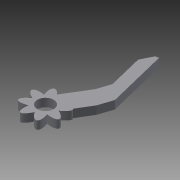
# Autodesk Inventor part: BrazoPinza
Saved by Autodesk Inventor 2015 (Build 190159000, 159)
## iProperties
Created: 2013-11-10
Part Number: BrazoPinza
Material: Genérico
Document SubType Name: Modeling
Designer: Gregorio
Density: 1 g/cm^3
Appearance: Valor por defecto
Author: Gregorio
Autodesk Inventor part; units mm, degrees
ref_plane "YZ Plane" through (0, 0, 0) normal (1, 0, 0) x (0, 1, 0)
ref_plane "XZ Plane" through (0, 0, 0) normal (0, 1, 0) x (-1, 0, 0)
ref_plane "XY Plane" through (0, 0, 0) normal (0, 0, 1) x (1, 0, 0)
sketch "Boceto1" plane through (0, 0, 0) normal (0, 0, 1) x (1, 0, 0)
  circle A0 centre (0, 0) radius 12.5
  circle A1 centre (0, 0) radius 4
  ellipse E0 centre (0, 4) end of major axis (0, 12.5) minor radius 3
  ellipse E1 centre (2.85, 2.8067) end of major axis (8.9175, 8.7595) minor radius 3
  ellipse E2 centre (4, 0) end of major axis (12.5, 0) minor radius 3
  ellipse E3 centre (2.85, -2.8067) end of major axis (8.8031, -8.8744) minor radius 3
  ellipse E4 centre (0, -4) end of major axis (0, -12.5) minor radius 3
  ellipse E5 centre (-2.85, -2.8067) end of major axis (-8.9175, -8.7595) minor radius 3
  ellipse E6 centre (-4, 0) end of major axis (-12.5, 0) minor radius 3
  ellipse E7 centre (-2.85, 2.8067) end of major axis (-8.8031, 8.8744) minor radius 3
  dimension "d1" = 8
  dimension "d4" = 3
  dimension "d5" = 3
  dimension "d6" = 3
  dimension "d7" = 3
  dimension "d8" = 3
  dimension "d9" = 3
  dimension "d10" = 3
  dimension "d11" = 3
  dimension "d0" = 25
  dimension "d12" = 2.85
  dimension "d14" = 2.85
  dimension "d15" = 2.85
  dimension "d16" = 2.85
  constraints: 2 coincident, 2 horizontal alignment, 2 vertical alignment, 1 centre point, 34 other
  measures "d0" diameter of A0
  measures "d12" horizontal distance of point (2.85, 2.807) point (0, 4)
  measures "d14" horizontal distance of point (-2.85, 2.807) point (0, 4)
  measures "d15" horizontal distance of point (0, -4) point (-2.85, -2.807)
  measures "d16" horizontal distance of point (2.85, -2.807) point (0, -4)
extrude "Extrusión1" add sketch "Boceto1" along normal blind 2 contours E2 E3 E6 E1 | E1 E2 E5 E0 | E3 E4 E7 E2 | E1 E6 A1 E5 E2 | E2 E7 A1 E6 E3 | E0 E1 E4 E7 | E0 E5 A1 E4 E1 | E4 E5 E0 E3 | E3 E0 A1 E7 E4 | E6 E3 E1 | E1 E3 A1 E6 | E5 A1 E0 E2 | E2 E0 E5 | E7 E4 E2 | E2 E4 A1 E7 | E6 A1 E1 E3 | E7 E0 E3 E6 | E7 E4 A1 E3 E0 | E0 E2 A1 E5 | E4 A1 E7 E1 | E1 E7 E4 | E5 E6 E1 E4 | E4 E1 A1 E0 E5 | E3 E5 A1 E0 | E0 E5 E3 | E7 A1 E2 E4 | E1 A1 E3 | E6 E5 A1 | A1 E3 E5 E6 | E0 A1 E2 | E5 E6 E0 A1 | E2 A1 E4 | E7 E6 A1 | A1 E4 E6 E7 | E6 E7 E1 A1 | E6 E7 E2 E5 | E6 E3 A1 E2 E7 | E3 A1 E6 E0 | E0 E6 E3 | E7 E1 A1 E4 | E5 E4 A1 | A1 E2 E4 E5 | E7 A1 E1 | E4 E5 E7 A1 | E5 E2 A1 E1 E6 | E4 E6 A1 E1 | E1 E6 E4 | E0 A1 E3 E5 | E0 E7 A1 | A1 E5 E7 E0 | E3 A1 E5 | E7 E0 E2 A1 | E1 E7 E5 E3 A1 | E5 E3 E0 E6 | E0 E6 E4 E2 A1 | E2 E0 E6 E4 A1 | E6 E4 E1 E7 | E6 E0 A1 E3 | E7 E5 E2 | E2 A1 E5 E7 | E6 A1 E0 | E3 E4 E6 A1 | A1 E4 E3 | A1 E1 E3 E4 | E4 E2 E7 E5 | A1 E7 E5 E3 E1 | E5 E7 A1 E2 | E1 A1 E4 E6 | E1 E0 A1 | A1 E6 E0 E1 | E4 A1 E6 | E0 E1 E3 A1 | A1 E3 E1 E7 E5 | E7 E5 E2 E0 | E1 E4 E5 E7 | E5 E7 E0 E3 | E0 E3 E4 E6 | E4 E6 E7 E2 | E2 E5 E6 E0 | E6 E0 E1 E4 | E3 E2 A1 | A1 E0 E2 E3 | E2 E3 E5 A1 | E5 A1 E7 | A1 E6 E4 E2 E0 | E3 E1 E6 E4 | E7 E2 E3 E5 | E3 E5 E6 E1 | E2 E1 A1 | A1 E7 E1 E2 | E1 E2 E4 A1 | A1 E4 E2 E0 E6 | E0 E6 E3 E1 | E7 E1 E2 E5 | E3 E6 E7 E1 | E1 E0 E5 E4 | E5 E4 E0 E7 | E0 E7 E4 E3 | E4 E3 E7 E6 | E7 E6 E3 E2 | E6 E5 E1 E0 | E2 E1 E6 E5 | E2 E0 E5 E3 | E5 E3 E1 E7 A1 | E2 E4 E5 E0 | E6 E1 E2 E4 | E3 E2 E6 E5 | E6 E5 E2 E1 | E1 E7 E4 E2 | E0 E2 E3 E6 | E4 E7 E0 E2 | E7 E6 E2 E1 | E3 E2 E7 E6 | E1 E5 E0 | E5 E0 E4 | E0 E4 E7 | E4 E7 E3 | E7 E3 E6 | E3 E6 E2 | E6 E1 E5 | E2 E6 E1 | E5 E0 E1 E3 | E1 E3 E4 E7 | E5 E4 E1 E0 | E2 E1 E5 E4 | E6 E2 E5 | E2 E5 E1 | E0 E7 E3 E2 | E4 E3 E0 E7 | E7 E2 E6 | E3 E7 E2 | E5 E1 E6 E2 E7 E3 E0 E4 | E1 E0 E4 E3 | E1 E4 E0 | E5 E1 E4 | E0 E3 E7 | E4 E0 E3
sketch "Boceto8" plane through (0, 0, 2) normal (0, 0, 1) x (1, 0, 0)
  line L0 (5.1447, -3.0874) -> (-5.1284, 3.1144)
  line L1 (-5.1284, 3.1144) -> (10.376, 28.7973)
  line L2 (10.376, 28.7973) -> (20.6492, 22.5956)
  line L3 (20.6492, 22.5956) -> (5.1447, -3.0874)
  line L4 (-3.7155, 2.2614) -> (5, -3)
  point P0 (-0.9996, -4.2411)
  point P1 (0.9996, -4.2411)
  point P2 (3.724, 2.2639)
  point P3 (2.3202, 3.6872)
  point P4 (-2.3223, 3.696)
  dimension "d92" = 30
  dimension "d93" = 12
  constraints: 10 end point, 2 parallel, 1 collinear, 1 perpendicular
  measures "d92" distance of L0.end L1.end
  measures "d93" distance of L0.start L0.end
extrude "Extrusión7" add sketch "Boceto8" along normal blind 3
sketch "Boceto3" plane through (0, 0, 2) normal (0, 0, 1) x (1, 0, 0)
  circle A0 centre (0, 0) radius 5
  dimension "d19" = 10
  constraints: 1 centre point
  measures "d19" diameter of A0
extrude "Extrusión2" cut sketch "Boceto3" along normal mid plane 10
sketch "Boceto29" plane through (0, 0, 5) normal (0, 0, 1) x (1, 0, 0)
  line L0 (20.6492, 22.5956) -> (10.376, 28.7973) projected
  line L1 (20.6492, 22.5956) -> (18.9527, 29.4601)
  line L2 (18.9527, 29.4601) -> (48.0766, 36.6574)
  line L3 (48.0766, 36.6574) -> (49.773, 29.7929)
  line L4 (49.773, 29.7929) -> (20.6492, 22.5956)
  dimension "d94" = 30
  dimension "d98" = 45
  dimension "d99" = 5
  constraints: 8 end point, 2 parallel, 1 perpendicular
  measures "d94" distance of L1.end L2.end
  measures "d98" angle of L0 L1
  measures "d99" distance from line of L1.end L0
extrude "Extrusión26" add sketch "Boceto29" against normal blind 3
sketch "Boceto30" plane through (18.9527, 29.4601, 2) normal (-0.9707952, -0.2399099, 0) x (0, 0, 1)
  line L0 (3, 0) -> (3, -7.0711) projected
  line L1 (3, 0) -> (0, 0) projected
  line L2 (0, -7.0711) -> (0, 0) projected
  line L3 (0, -7.0711) -> (3, -7.0711) projected
  point P0 (-2, -24.0528)
extrude "Extrusión27" add sketch "Boceto30" along normal up to next
sketch "Boceto32" plane through (0, 0, 5) normal (0, 0, 1) x (1, 0, 0)
  line L0 (12.0882, 27.7637) -> (10.376, 28.7973) projected
  line L1 (10.376, 28.7973) -> (-5.1284, 3.1144) projected
  line L2 (12.0882, 27.7637) -> (8.6581, 31.0712)
  line L3 (8.6581, 31.0712) -> (2.4109, 24.5926)
  line L4 (2.4109, 24.5926) -> (5.841, 21.2851)
  line L5 (5.841, 21.2851) -> (12.0882, 27.7637)
  point P0 (3.5, 12.105)
  point P1 (-5.1284, 3.1144)
  dimension "d108" = 9
  constraints: 8 end point, 2 parallel, 1 perpendicular, 2 other
  measures "d108" distance of L2.end L3.end
extrude "Extrusión29" cut sketch "Boceto32" against normal blind 6
sketch "Boceto33" plane through (0, 0, 5) normal (0, 0, 1) x (1, 0, 0)
  line L0 (12.0882, 27.7637) -> (5.841, 21.2851) projected
  line L1 (5.1447, -3.0874) -> (20.6492, 22.5956) projected
  line L2 (20.6492, 22.5956) -> (49.773, 29.7929) projected
  line L3 (23.1492, 23.2134) -> (21.5266, 24.778)
  line L4 (21.5266, 24.778) -> (15.8387, 18.8794)
  line L5 (15.8387, 18.8794) -> (17.4612, 17.3148)
  line L6 (17.4612, 17.3148) -> (23.1492, 23.2134)
  point P0 (8.5, 0.0802)
  dimension "d111" = 2.5
  constraints: 8 end point, 3 parallel, 1 perpendicular, 1 point on line, 2 other
  measures "d111" horizontal distance of L3.start L2.start
extrude "Extrusión30" add sketch "Boceto33" against normal blind 3
mirror "Simetría4" about plane through (5.1447, -3.0874, 2) normal (0.8560978, -0.5168139, 0) remove original yes
sketch "Boceto34" plane through (10.2732, -6.2018, 2) normal (0, 0, 1) x (0.8560978, -0.5168139, 0)
  arc A0 (-5, 0.0158) -> (5, 0.0158) centre (0, 0) ccw projected
  line L0 (-6, 0.0158) -> (-5, 0.0158) projected
  line L1 (-6, 6.5847) -> (-6, 0.0158) projected
  ellipse E0 centre (-3.4244, 2.0673) end of major axis (3.8524, -2.3257) minor radius 3 (-6, 6.5847) -> (-7.3152, 1.1128) ccw projected
  ellipse E1 centre (-3.8904, -0.9299) end of major axis (4.3419, 1.1881) minor radius 3 (-7.3152, 1.1128) -> (-5.9482, -4.3774) ccw projected
  ellipse E2 centre (-2.0673, -3.4244) end of major axis (2.3257, 3.8524) minor radius 3 (-5.9482, -4.3774) -> (-1.0693, -7.2598) ccw projected
  ellipse E3 centre (0.9893, -3.8757) end of major axis (-1.1285, 4.3562) minor radius 3 (-1.0693, -7.2598) -> (4.4424, -5.977) ccw projected
  ellipse E4 centre (3.4244, -2.0673) end of major axis (-3.8524, 2.3257) minor radius 3 (4.4424, -5.977) -> (7.3152, -1.1128) ccw projected
  ellipse E5 centre (3.8904, 0.9299) end of major axis (-4.3419, -1.1881) minor radius 3 (7.3152, -1.1128) -> (6, 4.384) ccw projected
  line L2 (6, 0.0158) -> (6, 4.384) projected
  line L3 (5, 0.0158) -> (6, 0.0158) projected
  point P0 (-12, 0)
  constraints: 6 other
extrude "Extrusión31" add sketch "Boceto34" along normal blind 3
sketch "Boceto35" plane through (17.7327, -5.4548, 2) normal (0, 0, 1) x (0.8560978, -0.5168139, 0)
  line L0 (0, 0) -> (0, 6.3601) projected
  ellipse E0 centre (-3.9327, -1.0702) end of major axis (-8.3257, -8.3471) minor radius 3 (0, 0) -> (0, 6.3601) ccw projected
  point P0 (-18, -4.4946)
  constraints: 1 other
extrude "Extrusión32" add sketch "Boceto35" along normal blind 3
chamfer "Chaflán6" distance 5 angle 50 1 edges at (13.4519, 51.7194, 3.5) measured on face at (13.9373, 51.8394, 3.5)
sketch "Boceto36" plane through (8.5397, 2.5363, 2) normal (0, 0, -1) x (-0.8560978, 0.5168139, 0)
  line L0 (17.6777, 48.1798) -> (16.9997, 40.4307) projected
  line L1 (16.2132, 49.6442) -> (17.6777, 48.1798) projected
  line L2 (16.2132, 49.6442) -> (-10, 23.431) projected
  line L3 (-12, 14.6561) -> (-10, 23.431) projected
  line L4 (-12, 4.2699) -> (-12, 14.6561) projected
  ellipse E0 centre (-8.0673, -3.1604) end of major axis (-3.6743, -10.4372) minor radius 3 (-7.0693, 0.675) -> (-12, 4.2699) ccw projected
  ellipse E1 centre (-5.0107, -2.709) end of major axis (-7.1285, -10.941) minor radius 3 (-1.5576, -0.6078) -> (-7.0693, 0.675) ccw projected
  ellipse E2 centre (-2.5756, -4.5175) end of major axis (-9.8524, -8.9104) minor radius 3 (0, 0) -> (-1.5576, -0.6078) ccw projected
  line L5 (0, 17.2626) -> (0, 0) projected
  line L6 (1.8209, 25.252) -> (0, 17.2626) projected
  line L7 (16.9997, 40.4307) -> (1.8209, 25.252) projected
  point P0 (6, -6.5847)
  constraints: 3 other
extrude "Extrusión33" add sketch "Boceto36" along normal blind 2
